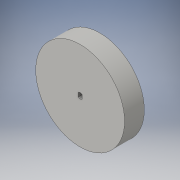
# Autodesk Inventor part: lazy susan platform
Saved by Autodesk Inventor 2016 (Build 200138000, 138)
## iProperties
Created: 2018-09-10
Part Number: lazy susan platform
Material: Generic
Document SubType Name: Modeling
Designer: student
Density: 1 g/cm^3
Appearance: Default
Author: student
Autodesk Inventor part; units mm, degrees
ref_plane "YZ Plane" through (0, 0, 0) normal (1, 0, 0) x (0, 1, 0)
ref_plane "XZ Plane" through (0, 0, 0) normal (0, 1, 0) x (-1, 0, 0)
ref_plane "XY Plane" through (0, 0, 0) normal (0, 0, 1) x (1, 0, 0)
sketch "Sketch1" plane through (0, 0, 0) normal (0, 0, 1) x (1, 0, 0)
  circle A0 centre (0, 0) radius 57.15
  line L0 (2.4402, 2.5908) -> (2.4402, -2.5908)
  line L1 (-2.4402, -2.5908) -> (-2.4402, 2.5908)
  line L2 (-2.4402, 2.5908) -> (2.4402, -2.5908) construction
  line L3 (2.4402, 2.5908) -> (-2.4402, -2.5908) construction
  arc A1 (2.4402, 2.5908) -> (-2.4402, 2.5908) centre (0, -0.0111) ccw
  arc A2 (-2.4402, -2.5908) -> (2.4402, -2.5908) centre (0, -0.0696) ccw
  dimension "d0" = 114.3
  dimension "d1" = 5.1816
  dimension "d2" = 4.8803
  dimension "d5" = 3.5671
  constraints: 8 end point, 4 point on circle, 3 centre point, 2 midpoint, 1 coincident, 1 parallel
  measures "d0" diameter of A0
  measures "d1" distance of L0.start L0.end
  measures "d2" distance between parallel lines of L0 L1
  measures "d5" radius of A1
extrude "Extrusion2" add sketch "Sketch1" along normal blind 25.4
body "Solid2"
